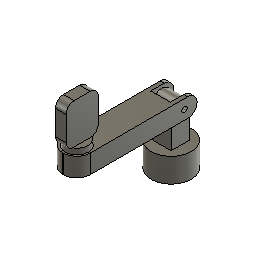
Crank_v4 (Autodesk Fusion 360 design; units mm, degrees)
Autodesk Fusion 360 part; units mm, degrees
sketch "Sketch1" plane through (0, 0, 0) normal (1, 0, 0) x (0, 0, -1)
  line L0 (0, 0) -> (7, 0)
  line L1 (7, 0) -> (7, -15)
  line L2 (7, -15) -> (0, -15)
  line L3 (0, -15) -> (0, 0)
  circle A0 centre (3.5, -2.606) radius 1
  dimension "d1" = 7
  dimension "d2" = 15
  dimension "d3" = 2
  constraint horizontal L0
  constraint vertical L1
  constraint horizontal L2
  constraint vertical L3
  constraint coincident L0.start L3.end
  measures "d1" distance of L0.start L0.end
  measures "d2" distance of L0.start L2.end
  measures "d3" diameter of A0
  measures "d78" distance of L0.end
extrude "Extrude1" add sketch "Sketch1" along normal blind 7 makes body 1
fillet "Fillet1" radius 3.5 2 edges at (3.5, 0, -7) (3.5, 0, 0) on bodies 1
sketch "Sketch2" plane through (0, -15, 0) normal (0, -1, 0) x (1, 0, 0)
  line L0 (0, 0) -> (0, -7)
  line L1 (0, -7) -> (7, -7)
  line L2 (7, -7) -> (7, 0)
  line L3 (7, 0) -> (0, 0)
  circle A0 centre (3.5, -3.5) radius 1.5
  dimension "d7" = 3
  dimension "d8" = 3.5
  dimension "d9" = 3.5
  measures "d7" diameter of A0
  measures "d8" distance of L2 A0.centre
  measures "d9" distance of L3 A0.centre
extrude "Extrude2" cut sketch "Sketch2" against normal blind 10 contours A0 bodies 1
copy_body "Body->Comp1" bodies 1 removing the originals makes body 2 in component "BodyConnector"
sketch "Sketch3" plane through (0, 0, 0) normal (0, 1, 0) x (1, 0, 0)
  circle A0 centre (5, -5) radius 7.5
  circle A1 centre (5, -5) radius 1.875
  circle A2 centre (5, -5) radius 3
  dimension "d12" = 3.75
  dimension "d13" = 6
  dimension "d19" = 15
  constraint concentric A0 A1
  constraint concentric A0 A2
  measures "d12" diameter of A1
  measures "d13" diameter of A2
  measures "d19" diameter of A0
extrude "Extrude3" add sketch "Sketch3" along normal blind 4 separate body contours A0 makes body 3
extrude "Extrude4" add sketch "Sketch3" along normal blind 5 from surface at 4 contours A0 | A2 bodies 3
copy_body "Body->Comp2" bodies 3 removing the originals makes body 4 in component "BodyAnchor"
ref_plane "WorkPlane1" through (5, 9, 5) normal (0, 1, 0) x (0, 0, 1) in component "BodyAnchor"
sketch "Sketch4" plane through (0, 0, 0) normal (0, 1, 0) x (1, 0, 0)
  line L0 (-2.3, -7) -> (-2.3, -52)
  line L1 (-2.3, -52) -> (8, -52)
  line L2 (8, -52) -> (8, -7)
  line L3 (8, -7) -> (6.5, -7)
  line L4 (6.5, -7) -> (6.5, -15.5)
  line L5 (6.5, -15.5) -> (-0.8, -15.5)
  line L6 (-0.8, -15.5) -> (-0.8, -7)
  line L7 (-0.8, -7) -> (-2.3, -7)
  dimension "d36" = 7.3
  dimension "d37" = 1.5
  dimension "d38" = 45
  dimension "d39" = 8.5
  constraint vertical L0
  constraint perpendicular L0 L1
  constraint perpendicular L1 L2
  constraint perpendicular L2 L3
  constraint perpendicular L3 L4
  constraint perpendicular L2 L5
  constraint perpendicular L5 L6
  constraint perpendicular L0 L7
  constraint equal L3 L7
  measures "d36" distance of L4.end L5.end
  measures "d37" distance of L2 L4
  measures "d38" distance of L0.start L0.end
  measures "d39" distance of L3.end L4.end
extrude "Extrude5" add sketch "Sketch4" along normal blind 7 separate body makes body 5
sketch "Sketch5" plane through (8, 0, 0) normal (1, 0, 0) x (0, 0, -1)
  line L0 (-52, 0) -> (-7, 0)
  line L1 (-7, 0) -> (-7, 7)
  line L2 (-7, 7) -> (-52, 7)
  line L3 (-52, 7) -> (-52, 0)
  circle A0 centre (-11.7, 3.5) radius 1
  dimension "d42" = 2
  dimension "d43" = 4.7
  dimension "d44" = 3.5
  measures "d42" diameter of A0
  measures "d43" distance of L1 A0.centre
  measures "d44" distance of L0 A0.centre
extrude "Extrude6" cut sketch "Sketch5" against normal up to surface (10.3 mm away) contours A0 bodies 5
copy_body "Body->Comp3" bodies 5 removing the originals makes body 6 in component "CrankShaft"
fillet "Fillet1'" radius 5 2 edges at (-2.3, 3.5, 52) (8, 3.5, 52) on bodies 6 in component "CrankShaft"
sketch "Sketch6" plane through (0, 0.894, 0.1) normal (0, 1, 0) x (-1, 0, 0)
  arc A0 (-3.5, 36.7) -> (-8.5, 31.7) centre (-3.5, 31.7) ccw
  line L0 (-8.5, 31.7) -> (-8.5, -8.3)
  line L1 (-8.5, -8.3) -> (-7, -8.3)
  line L2 (-7, -8.3) -> (-7, 0.2)
  line L3 (-7, 0.2) -> (0.3, 0.2)
  line L4 (0.3, 0.2) -> (0.3, -8.3)
  line L5 (0.3, -8.3) -> (1.8, -8.3)
  line L6 (1.8, -8.3) -> (1.8, 31.7)
  arc A1 (1.8, 31.7) -> (-3.2, 36.7) centre (-3.2, 31.7) ccw
  circle A2 centre (-3.5, 31.7) radius 4.35
  circle A3 centre (-3.5, 31.7) radius 1.75
  circle A4 centre (-3.5, 31.7) radius 2.75
  line L7 (-3.2, 36.7) -> (-3.5, 36.7)
  dimension "d60" = 8.7
  dimension "d63" = 3.5
  dimension "d64" = 5.5
  constraint concentric A0 A2
  constraint concentric A0 A3
  constraint concentric A0 A4
  measures "d60" diameter of A2
  measures "d63" diameter of A3
  measures "d64" diameter of A4
extrude "Extrude2'" cut sketch "Sketch6" against normal up to surface (7 mm away) contours A3 sketch seen with x (1, 0, 0) y (0, 1, 0) z (0, 0, 1) at (-0.5, 6.106, 15.2) bodies 6 in component "CrankShaft"
extrude "Extrude1'" cut sketch "Sketch6" against normal blind 3 contours A2 | A3 | A4 sketch seen with x (1, 0, 0) y (0, 1, 0) z (0, 0, 1) at (-0.5, 6.106, 15.2) bodies 6 in component "CrankShaft"
extrude "Extrude3'" cut sketch "Sketch6" along normal blind 3 from surface at -7 contours A3 | A4 sketch seen with x (1, 0, 0) y (0, 1, 0) z (0, 0, 1) at (-0.5, 6.106, 15.2) bodies 6 in component "CrankShaft"
ref_plane "WorkPlane1" through (3.5, -2.606, 14.3) normal (1, 0, 0) x (0, 0, -1)
sketch "Sketch7" plane through (0, 0, 0) normal (0, 1, 0) x (1, 0, 0)
  circle A0 centre (22.2122, -15.8104) radius 4.125
  line L0 (20.2122, -9.8104) -> (24.2122, -9.8104)
  line L1 (24.2122, -9.8104) -> (24.2122, -21.8104)
  line L2 (24.2122, -21.8104) -> (20.2122, -21.8104)
  line L3 (20.2122, -21.8104) -> (20.2122, -9.8104)
  circle A1 centre (22.2122, -15.8104) radius 1.5
  line L4 (22.2122, -9.8104) -> (22.2122, -15.8104) construction
  line L5 (22.2122, -15.8104) -> (22.2122, -21.8104) construction
  line L6 (22.2122, -15.8104) -> (24.2122, -15.8104) construction
  line L7 (22.2122, -15.8104) -> (20.2122, -15.8104) construction
  dimension "d71" = 8.25
  dimension "d77" = 3
  dimension "d78" = 12
  dimension "d79" = 4
  constraint horizontal L0
  constraint vertical L1
  constraint horizontal L2
  constraint vertical L3
  constraint concentric A0 A1
  constraint midpoint L0 L4.start
  constraint coincident A0.centre A1.centre
  constraint midpoint L2 L5.end
  constraint midpoint L1 L6.end
  constraint midpoint L3 L7.end
  constraint equal L6 L7
  constraint equal L4 L5
  measures "d71" diameter of A0
  measures "d77" diameter of A1
  measures "d78" distance of L0.end L1.end
  measures "d79" distance of L0.start L0.end
extrude "Extrude1''" add sketch "Sketch7" along normal blind 5 separate body contours A0 L1 | A0 L1 L3 | A0 L3 | A1 makes body 7 in component "Handle"
extrude "Extrude2''" add sketch "Sketch7" along normal blind 15 from surface at 5 contours A0 L1 L3 | A0 L0 L1 L3 | A0 L1 L2 L3 | A1 bodies 7 in component "Handle"
extrude "Extrude3''" cut sketch "Sketch7" along normal blind 4 contours A1 bodies 7 in component "Handle"
fillet "Fillet2" radius 3.5 4 edges at (7.25, 7, 7) (-1.55, 7, 7) (7.25, 0, 7) (-1.55, 0, 7) on bodies 6 in component "CrankShaft"
fillet "Fillet6" radius 3 4 edges at (22.2122, 5, 21.8104) (22.2122, 20, 21.8104) (22.2122, 20, 9.8104) (22.2122, 5, 9.8104) on bodies 7 in component "Handle"
component "BodyConnector" placed x (1, 0, 0) y (0, 1, 0) z (0, 0, 1) at (0, 0, 0)
component "BodyAnchor" placed x (1, 0, 0) y (0, 1, 0) z (0, 0, 1) at (-1.5, -24, -8.5)
component "CrankShaft" placed x (1, 0, 0) y (0, 1, 0) z (0, 0, 1) at (0.5, -6.106, -15.2)
component "Handle" placed x (1, 0, 0) y (0, 1, 0) z (0, 0, 1) at (-18.7122, -2.106, 15.9896)
equation "d1 = baseWid"
equation "d2 = baseHei"
equation "d3 = dFilament"
equation "d4 = baseWid"
equation "baseWid = 7 mm"
equation "baseHei = 15 mm"
equation "dFilament = 2 mm"
equation "d36 = baseWid + 0.3 mm"
equation "d39 = baseWid + 1.5 mm"
equation "d40 = baseWid"
equation "d42 = dFilament"
equation "d43 = baseWid - ( 0.9 mm + ( dFilament / 2 ) + 0.4 mm )"
equation "d44 = baseWid / 2"
